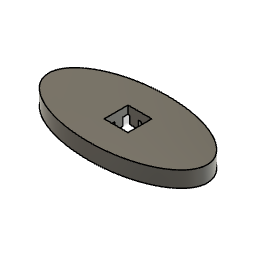
assy (Autodesk Fusion 360 archive; units mm, degrees)
design "cam gear"
Autodesk Fusion 360 part; units mm, degrees
sketch "Sketch1" plane through (0, 0, 0) normal (0, 1, 0) x (1, 0, 0)
  ellipse E0 centre (0, 0) end of major axis (10, 0) minor radius 5
  line L0 (-10, 0) -> (10, 0)
  line L1 (0, -5) -> (0, 5)
  line L2 (1.5, -1.5) -> (-1.5, -1.5)
  line L3 (-1.5, -1.5) -> (-1.5, 1.5)
  line L4 (-1.5, 1.5) -> (1.5, 1.5)
  line L5 (1.5, 1.5) -> (1.5, -1.5)
  line L6 (1.5, -1.5) -> (-1.5, 1.5) construction
  line L7 (-1.5, -1.5) -> (1.5, 1.5) construction
  dimension "d1" = 10
  dimension "d2" = 5
  dimension "d3" = 3
  dimension "d4" = 3
  constraint coincident E0.centre origin
  constraint horizontal L0
  constraint coincident E0 L0.start
  constraint coincident E0 L0.end
  constraint coincident E0 L1.start
  constraint coincident E0 L1.end
  constraint horizontal L2
  constraint perpendicular L2 L3
  constraint parallel L2 L4
  constraint parallel L3 L5
  constraint coincident L6 E0.centre
  constraint coincident L7 E0.centre
  measures "d1" distance of E0.centre L0.end
  measures "d2" distance of E0.centre L1.end
  measures "d3" distance of L3.end L4.end
  measures "d4" distance of L2.end L3.end
extrude "Extrude1" add sketch "Sketch1" along normal blind 2 contours E0 L0 L1 L4 L5 | E0 L0 L1 L2 L5 | E0 L0 L1 L3 L4 | E0 L0 L1 L2 L3 makes body 1
sketch "Sketch2" plane through (0, 0, 0) normal (0, -1, 0) x (1, 0, 0)
  line L0 (1.5, -1.5) -> (-1.5, -1.5)
  line L1 (-1.5, -1.5) -> (-1.5, 1.5)
  line L2 (-1.5, 1.5) -> (1.5, 1.5)
  line L3 (1.5, 1.5) -> (1.5, -1.5)
  ellipse E0 centre (0, 0) end of major axis (10, 0) minor radius 5 construction
  spline S0 degree 3 poles (-9, 0) (-9, -0.4805) (-8.7749, -1.0144) (-8.1755, -1.5893) (-7.3375, -2.3933) (-5.7684, -3.165) (-3.8472, -3.5923) (-1.5715, -4.0984) (1.1676, -4.1273) (3.4888, -3.6676) (5.2672, -3.3153) (6.7888, -2.6785) (7.7397, -1.9591) (8.5093, -1.3767) (8.8839, -0.7763) (8.9752, -0.2732) (9.0582, 0.1847) (8.958, 0.6291) (8.5638, 1.155) (8.019, 1.8817) (6.848, 2.6682) (5.2592, 3.2021) (3.1557, 3.9089) (0.3632, 4.1706) (-2.1616, 3.8753) (-4.2224, 3.6343) (-6.0882, 3.0261) (-7.3018, 2.261) (-8.2243, 1.6794) (-8.7451, 1.0304) (-8.9198, 0.492) (-8.9749, 0.3222) (-9, 0.1608) (-9, 0) knots -3.141593 -3.141593 -3.141593 -3.141593 -2.661128 -2.661128 -2.661128 -1.989339 -1.989339 -1.989339 -1.193608 -1.193608 -1.193608 -0.583919 -0.583919 -0.583919 -0.090453 -0.090453 -0.090453 0.358594 0.358594 0.358594 0.979103 0.979103 0.979103 1.800593 1.800593 1.800593 2.471093 2.471093 2.471093 2.980773 2.980773 2.980773 3.141593 3.141593 3.141593 3.141593
  line L4 (-0.5, 1.5) -> (-0.5, 3.9898)
  line L5 (0.5, 1.5) -> (0.5, 3.9898)
  line L6 (-1.079, 1.5) -> (-3.7306, 3.6146)
  line L7 (-1.4845, 0.5443) -> (-4.939, 3.2992)
  line L8 (-1.5, 0.1705) -> (-8.3644, -1.3963)
  line L9 (-1.5, -0.8552) -> (-7.3883, -2.1992)
  line L10 (-1.2773, -1.5) -> (-2.4053, -3.8422)
  line L11 (-0.1674, -1.5) -> (-1.3455, -3.9464)
  line L12 (0.1674, -1.5) -> (1.346, -3.9473)
  line L13 (1.2773, -1.5) -> (2.4058, -3.8432)
  line L14 (1.5, -0.8552) -> (7.3943, -2.2006)
  line L15 (1.5, 0.1705) -> (8.3629, -1.3959)
  line L16 (1.4845, 0.5443) -> (4.9439, 3.3031)
  line L17 (1.079, 1.5) -> (3.7295, 3.6137)
  dimension "d7" = -1
  constraint coincident L2 L4.start
  constraint coincident S0 L4.end
  constraint perpendicular L2 L4
  constraint coincident S0 L6.end
  constraint coincident S0 L7.end
  constraint coincident S0 L8.end
  constraint coincident S0 L10.end
  constraint coincident S0 L11.end
  constraint coincident S0 L9.end
  constraint coincident S0 L12.end
  constraint coincident S0 L13.end
  constraint coincident S0 L14.end
  constraint coincident S0 L15.end
  constraint coincident S0 L16.end
  constraint coincident S0 L17.end
  constraint coincident L1 L9.start
  constraint coincident L2 L6.start
  constraint coincident L2 L17.start
  constraint coincident L3 L14.start
  constraint coincident L0 L13.start
  constraint coincident L0 L10.start
  constraint coincident L1 L8.start
  constraint coincident L0 L11.start
  constraint coincident L0 L12.start
  constraint coincident L3 L15.start
extrude "Extrude2" cut sketch "Sketch2" against normal blind 1 contours L0 L3 S0 L13 L14 | L0 S0 L11 L12 | L3 S0 L15 L16 | L0 L1 S0 L9 L10 | L2 S0 L5 L17 | L1 S0 L7 L8 | L2 S0 L4 L6 bodies 1
copy_body "Body->Comp1" bodies 1 removing the originals makes body 2 in component "Component"
component "Component" placed x (1, 0, 0) y (0, 1, 0) z (0, 0, 1) at (0, 0, 0)

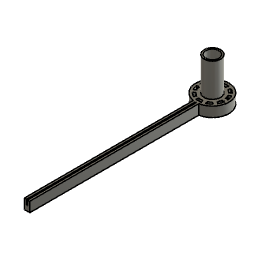
design "reciprocator"
Autodesk Fusion 360 part; units mm, degrees
sketch "Sketch1" plane through (0, 0, 0) normal (0, 1, 0) x (1, 0, 0)
  circle A0 centre (0, 0) radius 5
  circle A1 centre (0, 0) radius 2.5
  line L0 (-4.9749, -0.5) -> (-4.9749, 0.5)
  line L1 (4.9749, 0.5) -> (4.9749, -0.5)
  line L2 (-4.9749, 0.5) -> (-3.4641, 0.5)
  line L3 (3.4641, 0.5) -> (4.9749, 0.5)
  line L4 (4.9749, -0.5) -> (3.4641, -0.5)
  line L5 (-3.4641, -0.5) -> (-4.9749, -0.5)
  circle A2 centre (0, 0) radius 3.5
  line L6 (-0.5949, -3.4491) -> (-1.0618, -4.886)
  line L7 (-2.0129, -4.5769) -> (-1.546, -3.14)
  line L8 (2.0129, 4.5769) -> (1.546, 3.14)
  line L9 (0.5949, 3.4491) -> (1.0618, 4.886)
  line L10 (3.0964, -1.6316) -> (4.3187, -2.5197)
  line L11 (3.7309, -3.3287) -> (2.5086, -2.4407)
  line L12 (-3.7309, 3.3287) -> (-2.5086, 2.4407)
  line L13 (-3.0964, 1.6316) -> (-4.3187, 2.5197)
  line L14 (2.5086, 2.4407) -> (3.7309, 3.3287)
  line L15 (4.3187, 2.5197) -> (3.0964, 1.6316)
  line L16 (-4.3187, -2.5197) -> (-3.0964, -1.6316)
  line L17 (-2.5086, -2.4407) -> (-3.7309, -3.3287)
  line L18 (-1.546, 3.14) -> (-2.0129, 4.5769)
  line L19 (-1.0618, 4.886) -> (-0.5949, 3.4491)
  line L20 (1.0618, -4.886) -> (0.5949, -3.4491)
  line L21 (1.546, -3.14) -> (2.0129, -4.5769)
  arc A3 (-1.7794, 3.8585) -> (-3.1198, 2.8847) centre (0, 0) ccw
  arc A4 (-3.7076, 2.0757) -> (-4.2195, 0.5) centre (0, 0) ccw
  arc A5 (-4.2195, -0.5) -> (-3.7076, -2.0757) centre (0, 0) ccw
  arc A6 (-3.1198, -2.8847) -> (-1.7794, -3.8585) centre (0, 0) ccw
  arc A7 (-0.8284, -4.1675) -> (0.8284, -4.1675) centre (0, 0) ccw
  arc A8 (1.7794, -3.8585) -> (3.1198, -2.8847) centre (0, 0) ccw
  arc A9 (3.7076, -2.0757) -> (4.2195, -0.5) centre (0, 0) ccw
  arc A10 (4.2195, 0.5) -> (3.7076, 2.0757) centre (0, 0) ccw
  arc A11 (3.1198, 2.8847) -> (1.7794, 3.8585) centre (0, 0) ccw
  arc A12 (0.8284, 4.1675) -> (-0.8284, 4.1675) centre (0, 0) ccw
  line L22 (-0.8284, -5.9767) -> (-0.8284, -4.9309)
  line L23 (0.8284, -4.9309) -> (0.8284, -5.9767)
  line L24 (0.8284, -5.9767) -> (0.8284, -55.9767)
  line L25 (-0.8284, -5.9767) -> (-0.8284, -55.9767)
  line L26 (0.8284, -55.9767) -> (-0.8284, -55.9767)
  line L27 (0.1716, -5.9767) -> (0.1716, -55.9767)
  line L28 (0.1716, -5.9767) -> (0.1716, -4.9309)
  line L29 (-0.1716, -4.9309) -> (-0.1716, -5.9767)
  line L30 (-0.1716, -5.9767) -> (-0.1716, -55.9767)
  dimension "d1" = 10
  dimension "d2" = 5
  dimension "d10" = 1
  dimension "d11" = 1
  dimension "d13" = 360
  dimension "d16" = 1.0458
  dimension "d17" = 50
  dimension "d18" = 50
  constraint concentric A0 A1
  constraint horizontal L4
  constraint perpendicular L0 L4
  constraint parallel L2 L4
  constraint parallel L0 L1
  constraint coincident A0 L1.end
  constraint coincident A0.centre A1.centre
  constraint collinear L2 L3
  constraint collinear L4 L5
  constraint concentric A1 A2
  constraint coincident A2 L2.end
  constraint coincident A2 L5.start
  constraint coincident A2 L4.end
  constraint coincident A2 L3.start
  constraint concentric A1 A3
  constraint coincident L19 A12.end
  constraint coincident L18 A3.start
  constraint coincident L12 A3.end
  constraint coincident L13 A4.start
  constraint concentric A3 A4
  constraint coincident L2 A4.end
  constraint coincident L5 A5.start
  constraint concentric A4 A5
  constraint coincident L16 A5.end
  constraint coincident L17 A6.start
  constraint concentric A5 A6
  constraint coincident L7 A6.end
  constraint coincident L6 A7.start
  constraint concentric A6 A7
  constraint coincident L20 A7.end
  constraint coincident L21 A8.start
  constraint concentric A7 A8
  constraint coincident L11 A8.end
  constraint coincident L10 A9.start
  constraint concentric A8 A9
  constraint coincident L4 A9.end
  constraint coincident L3 A10.start
  constraint concentric A9 A10
  constraint coincident L15 A10.end
  constraint coincident L14 A11.start
  constraint concentric A10 A11
  constraint coincident L8 A11.end
  constraint coincident L9 A12.start
  constraint concentric A11 A12
  constraint parallel L22 L23
  constraint coincident A0 L23.start
  constraint coincident A0 L22.end
  constraint parallel L23 L24
  constraint parallel L22 L25
  constraint perpendicular L25 L26
  constraint parallel L25 L27
  constraint parallel L22 L28
  constraint parallel L23 L29
  constraint parallel L24 L30
  constraint coincident L26 L27.end
  constraint coincident L26 L30.end
  measures "d1" diameter of A0
  measures "d2" diameter of A1
  measures "d10" distance of L2 L4
  measures "d11" distance of A1 A2
  measures "d16" distance of L23.end L23.start
  measures "d17" distance of L23.end L24.end
  measures "d18" distance of L22.start L25.end
extrude "Extrude1" add sketch "Sketch1" along normal blind 10 contours A1 makes body 1
extrude "Extrude2" add sketch "Sketch1" against normal blind 3 separate body contours A0 L1 | A0 L3 L15 A10 | L1 L3 L4 A2 | A0 L4 L10 A9 | A0 A2 L14 L15 | L3 A2 L15 A10 | A0 A2 L10 L11 | L4 A2 L10 A9 | A0 L8 L14 A11 | A2 | A0 L11 L21 A8 | A0 A2 L8 L9 | A2 L8 L14 A11 | A0 A2 L20 L21 | A2 L11 L21 A8 | A0 L9 L19 A12 | A0 L6 L20 A7 | A0 A2 L18 L19 | A2 L9 L19 A12 | A2 L6 L20 A7 | A0 L12 L18 A3 | A0 A2 L6 L7 | A0 A2 L12 L13 | A2 L12 L18 A3 | A0 L2 L13 A4 | A2 L7 L17 A6 | A0 L7 L17 A6 | A0 L0 | L0 L2 L5 A2 | L2 A2 L13 A4 | A0 A2 L16 L17 | A0 L5 L16 A5 | L5 A2 L16 A5 makes body 2
sketch "Sketch2" plane through (0, 10, 0) normal (0, 1, 0) x (-1, 0, 0)
  circle A0 centre (0, 0) radius 2.5
  circle A1 centre (0, 0) radius 2
  dimension "d7" = 4
  constraint coincident A0.centre A1.centre
  measures "d7" diameter of A1
extrude "Extrude3" cut sketch "Sketch2" against normal blind 9 contours A1 bodies 1
extrude "Extrude4" cut sketch "Sketch1" against normal blind 3 contours L3 A2 L15 A10 | L4 A2 L10 A9 | A2 L8 L14 A11 | A2 L11 L21 A8 | A2 L9 L19 A12 | A2 L6 L20 A7 | A2 L12 L18 A3 | A2 L7 L17 A6 | L2 A2 L13 A4 | L5 A2 L16 A5 bodies 2
extrude "Extrude5" add sketch "Sketch1" against normal blind 3 contours A0 L23 L24 L26 L27 L28 | A0 L26 L27 L28 L29 L30 | A0 L22 L25 L26 L29 L30 bodies 2
extrude "Extrude6" cut sketch "Sketch1" against normal blind 1.5 contours A0 L26 L27 L28 L29 L30 bodies 2
combine "Combine1" operation add target body 2 tool bodies 1
copy_body "Body->Comp3" bodies 2 removing the originals makes body 3 in component "Component"
component "Component" placed x (1, 0, 0) y (0, 1, 0) z (0, 0, 1) at (0, 0, 0)

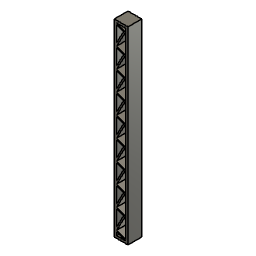
design "spindle"
Autodesk Fusion 360 part; units mm, degrees
sketch "Sketch1" plane through (0, 0, 0) normal (0, 1, 0) x (1, 0, 0)
  line L0 (1.45, -1.45) -> (-1.45, -1.45)
  line L1 (-1.45, -1.45) -> (-1.45, 1.45)
  line L2 (-1.45, 1.45) -> (1.45, 1.45)
  line L3 (1.45, 1.45) -> (1.45, -1.45)
  line L4 (1.45, -1.45) -> (-1.45, 1.45) construction
  line L5 (-1.45, -1.45) -> (1.45, 1.45) construction
  dimension "d1" = 2.9
  dimension "d2" = 2.9
  constraint horizontal L0
  constraint perpendicular L0 L1
  constraint parallel L0 L2
  constraint parallel L1 L3
  constraint coincident L4 origin
  constraint coincident L5 origin
  measures "d1" distance of L0.start L2.end
  measures "d2" distance of L1.end L2.end
extrude "Extrude1" add sketch "Sketch1" along normal blind 40 makes body 1
sketch "Sketch2" plane through (0, 0, 1.45) normal (0, 0, 1) x (1, 0, 0)
  line L0 (-1.45, 0) -> (1.45, 0)
  line L1 (1.45, 0) -> (1.45, 40)
  line L2 (1.45, 40) -> (-1.45, 40)
  line L3 (-1.45, 40) -> (-1.45, 0)
  line L4 (-0.95, 39.5) -> (-0.95, 0.5)
  line L5 (-0.95, 0.5) -> (0.95, 0.5)
  line L6 (0.95, 0.5) -> (0.95, 39.5)
  line L7 (0.95, 39.5) -> (-0.95, 39.5)
  line L8 (-0.95, 39.5) -> (0.95, 38.8085)
  line L9 (-0.95, 35.2778) -> (0.95, 34.5862)
  line L10 (-0.95, 31.0556) -> (0.95, 30.364)
  line L11 (-0.95, 26.8333) -> (0.95, 26.1418)
  line L12 (-0.95, 22.6111) -> (0.95, 21.9196)
  line L13 (-0.95, 18.3889) -> (0.95, 17.6973)
  line L14 (-0.95, 14.1667) -> (0.95, 13.4751)
  line L15 (-0.95, 9.9444) -> (0.95, 9.2529)
  line L16 (-0.95, 5.7222) -> (0.95, 5.0307)
  line L17 (-0.95, 1.5) -> (0.95, 0.8085)
  line L18 (0.95, 38.8085) -> (-0.95, 35.2778)
  line L19 (0.95, 34.5862) -> (-0.95, 31.0556)
  line L20 (0.95, 30.364) -> (-0.95, 26.8333)
  line L21 (0.95, 26.1418) -> (-0.95, 22.6111)
  line L22 (0.95, 21.9196) -> (-0.95, 18.3889)
  line L23 (0.95, 17.6973) -> (-0.95, 14.1667)
  line L24 (0.95, 13.4751) -> (-0.95, 9.9444)
  line L25 (0.95, 9.2529) -> (-0.95, 5.7222)
  line L26 (0.95, 5.0307) -> (-0.95, 1.5)
  line L27 (-1.0526, 39.2181) -> (0.5215, 38.6452)
  line L28 (0.5215, 38.6452) -> (-1.3785, 35.1145)
  line L29 (-1.3785, 35.1145) -> (0.5215, 34.423)
  line L30 (0.5215, 34.423) -> (-1.3785, 30.8923)
  line L31 (-1.3785, 30.8923) -> (0.5215, 30.2007)
  line L32 (0.5215, 30.2007) -> (-1.3785, 26.6701)
  line L33 (-1.3785, 26.6701) -> (0.5215, 25.9785)
  line L34 (0.5215, 25.9785) -> (-1.3785, 22.4478)
  line L35 (-1.3785, 22.4478) -> (0.5215, 21.7563)
  line L36 (0.5215, 21.7563) -> (-1.3785, 18.2256)
  line L37 (-1.3785, 18.2256) -> (0.5215, 17.5341)
  line L38 (0.5215, 17.5341) -> (-1.3785, 14.0034)
  line L39 (-1.3785, 14.0034) -> (0.5215, 13.3118)
  line L40 (0.5215, 13.3118) -> (-1.3785, 9.7812)
  line L41 (-1.3785, 9.7812) -> (0.5215, 9.0896)
  line L42 (0.5215, 9.0896) -> (-1.3785, 5.5589)
  line L43 (-1.3785, 5.5589) -> (0.5215, 4.8674)
  line L44 (0.5215, 4.8674) -> (-1.3785, 1.3367)
  line L45 (-1.3785, 1.3367) -> (0.9203, 0.5)
  dimension "d5" = -0.5
  dimension "d6" = 70
  dimension "d9" = -38
  dimension "d10" = 0
  constraint coincident L6 L8.end
  constraint parallel L8 L27
  constraint parallel L18 L28
  constraint parallel L9 L29
  constraint parallel L19 L30
  constraint parallel L10 L31
  constraint parallel L20 L32
  constraint parallel L11 L33
  constraint parallel L21 L34
  constraint parallel L12 L35
  constraint parallel L22 L36
  constraint parallel L13 L37
  constraint parallel L23 L38
  constraint parallel L14 L39
  constraint parallel L24 L40
  constraint parallel L15 L41
  constraint parallel L25 L42
  constraint parallel L16 L43
  constraint parallel L26 L44
  constraint parallel L17 L45
  constraint coincident L5 L45.end
  measures "d6" angle of L4 L8
extrude "Extrude2" cut sketch "Sketch2" against normal blind 2 contours L6 L7 L8 | L4 L27 L28 | L6 L9 L18 | L6 L10 L19 | L6 L11 L20 | L4 L29 L30 | L6 L12 L21 | L4 L31 L32 | L6 L13 L22 | L4 L33 L34 | L6 L14 L23 | L4 L35 L36 | L6 L15 L24 | L4 L37 L38 | L6 L16 L25 | L4 L39 L40 | L6 L17 L26 | L4 L41 L42 | L4 L43 L44 | L4 L5 L45 bodies 1
copy_body "Body->Comp1" bodies 1 removing the originals makes body 2 in component "Component"
component "Component" placed x (1, 0, 0) y (0, 1, 0) z (0, 0, 1) at (0, 0, 0)

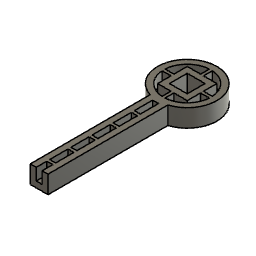
design "lever"
Autodesk Fusion 360 part; units mm, degrees
sketch "Sketch1" plane through (0, 0, 0) normal (0, 1, 0) x (1, 0, 0)
  circle A0 centre (0, 0) radius 5
  line L0 (1.5, -1.5) -> (-1.5, -1.5)
  line L1 (-1.5, -1.5) -> (-1.5, 1.5)
  line L2 (-1.5, 1.5) -> (1.5, 1.5)
  line L3 (1.5, 1.5) -> (1.5, -1.5)
  line L4 (1.5, -1.5) -> (-1.5, 1.5) construction
  line L5 (-1.5, -1.5) -> (1.5, 1.5) construction
  line L6 (0, 0) -> (0, -5) construction
  line L7 (1.5, -35) -> (-1.5, -35)
  line L8 (-1.5, 25) -> (1.5, 25)
  line L9 (0, -5) -> (-0.4988, 4.9751) construction
  line L10 (0, -5) -> (0.4988, 4.9751) construction
  line L11 (1.5, 1.5) -> (1.5, -1.5)
  line L12 (1.5, -4.7697) -> (1.5, -35)
  line L13 (-1.5, -35) -> (-1.5, -4.7697)
  line L14 (-1.5, -1.5) -> (-1.5, 1.5)
  dimension "d1" = 10
  dimension "d2" = 3
  dimension "d3" = 3
  dimension "d4" = 3
  dimension "d5" = 30
  constraint coincident A0.centre L6.start
  constraint horizontal L0
  constraint perpendicular L0 L1
  constraint parallel L0 L2
  constraint parallel L1 L3
  constraint coincident L4 A0.centre
  constraint coincident L5 A0.centre
  constraint perpendicular L0 L6
  constraint horizontal L7
  constraint perpendicular L7 L13
  constraint parallel L7 L8
  constraint parallel L11 L13
  constraint coincident A0 L6.end
  constraint coincident A0 L10.end
  constraint coincident A0 L9.end
  constraint coincident A0 L12.start
  constraint collinear L11 L12
  constraint coincident A0 L13.end
  constraint collinear L13 L14
  measures "d1" diameter of A0
  measures "d2" distance of L1.end L2.end
  measures "d3" distance of L0.start L2.end
  measures "d4" distance of L7.start L7.end
  measures "d5" distance of L7 L6.end
extrude "Extrude1" add sketch "Sketch1" along normal blind 3
sketch "Sketch2" plane through (0, 3, 0) normal (0, 1, 0) x (-1, 0, 0)
  line L0 (-1.5, 1.5) -> (1.5, 1.5)
  line L1 (1.5, 1.5) -> (1.5, -1.5)
  line L2 (1.5, -1.5) -> (-1.5, -1.5)
  line L3 (-1.5, -1.5) -> (-1.5, 1.5)
  arc A0 (-1.5, 4.7697) -> (1.5, 4.7697) centre (0, 0) ccw
  line L4 (1.5, 4.7697) -> (1.5, 35)
  line L5 (1.5, 35) -> (-1.5, 35)
  line L6 (-1.5, 35) -> (-1.5, 4.7697)
  line L7 (0.5, 34) -> (-0.5, 34)
  line L8 (-0.5, 34) -> (-0.5, 3.9686)
  arc A1 (0, 4) -> (0.2464, 3.9924) centre (0, 0) ccw
  line L9 (0.5, 3.9686) -> (0.5, 34)
  line L10 (-2.5, -2.5) -> (-2.5, 2.5)
  line L11 (-2.5, 2.5) -> (2.5, 2.5)
  line L12 (2.5, 2.5) -> (2.5, -2.5)
  line L13 (2.5, -2.5) -> (-2.5, -2.5)
  line L14 (-0.2536, -2.5) -> (-0.2536, -4)
  line L15 (0, -4) -> (0, -2.5) construction
  line L16 (0, -1.5) -> (0, 4.8511) construction
  line L17 (-0.2536, -4) -> (0, -2.5) construction
  line L18 (0.2464, -4) -> (0, -2.5) construction
  line L19 (0.2464, -4) -> (0.2464, -2.5)
  line L20 (2.5, -0.2536) -> (4, -0.2536)
  line L21 (4, 0.2464) -> (2.5, 0.2464)
  line L22 (0.2536, 2.5) -> (0.2536, 4)
  line L23 (-0.2464, 4) -> (-0.2464, 2.5)
  line L24 (-2.5, 0.2536) -> (-4, 0.2536)
  line L25 (-4, -0.2464) -> (-2.5, -0.2464)
  line L26 (0.5, 4.8511) -> (-0.5, 4.8511)
  line L27 (0.5, 5.3511) -> (-0.5, 5.3511)
  line L28 (0.5, 8.9225) -> (-0.5, 8.9225)
  line L29 (0.5, 8.4225) -> (-0.5, 8.4225)
  line L30 (0.5, 12.4939) -> (-0.5, 12.4939)
  line L31 (0.5, 11.9939) -> (-0.5, 11.9939)
  line L32 (0.5, 16.0654) -> (-0.5, 16.0654)
  line L33 (0.5, 15.5654) -> (-0.5, 15.5654)
  line L34 (0.5, 19.6368) -> (-0.5, 19.6368)
  line L35 (0.5, 19.1368) -> (-0.5, 19.1368)
  line L36 (0.5, 23.2082) -> (-0.5, 23.2082)
  line L37 (0.5, 22.7082) -> (-0.5, 22.7082)
  line L38 (0.5, 26.7796) -> (-0.5, 26.7796)
  line L39 (0.5, 26.2796) -> (-0.5, 26.2796)
  line L40 (0.5, 30.3511) -> (-0.5, 30.3511)
  line L41 (0.5, 29.8511) -> (-0.5, 29.8511)
  dimension "d9" = -1
  dimension "d12" = 0.5
  dimension "d14" = 360
  dimension "d15" = 0.5
  dimension "d18" = 0
  dimension "d19" = 0
  dimension "d22" = 25
  dimension "d23" = 0
  constraint perpendicular L11 L15
  constraint midpoint L13 L15.end
  constraint coincident L13 L14.start
  constraint coincident L2 L16.start
  constraint collinear L15 L16
  constraint coincident L13 L19.end
  constraint parallel L5 L7
  constraint parallel L6 L8
  constraint concentric A0 A1
  constraint parallel L4 L9
  constraint coincident A1 L15.start
  constraint coincident L9.start A1
  constraint coincident L8.end A1
  constraint coincident L9 L26.start
  constraint coincident L8 L26.end
  constraint perpendicular L8 L26
  constraint coincident L9 L27.start
  constraint coincident L8 L27.end
  constraint perpendicular L8 L27
  measures "d12" distance of L14 L19
  measures "d15" distance of L26 L27
extrude "Extrude3" cut sketch "Sketch2" against normal blind 2 contours L7 L8 L9 L40 | L8 L9 L38 L41 | L8 L9 L36 L39 | L8 L9 L34 L37 | L8 L9 L32 L35 | L8 L9 L30 L33 | L8 L9 L28 L31 | L8 L9 L27 L29 | A1 L11 L12 L21 L22 | A1 L10 L11 L23 L24 | A1 L12 L13 L19 L20 | A1 L10 L13 L14 L25
extrude "Extrude2" cut sketch "Sketch2" against normal blind 2 contours L7 L8 L9 L40 | L8 L9 L40 L41 | L8 L9 L38 L41 | L8 L9 L38 L39 | L8 L9 L36 L39 | L8 L9 L36 L37 | L8 L9 L34 L37 | L8 L9 L34 L35 | L8 L9 L32 L35 | L8 L9 L32 L33 | L8 L9 L30 L33 | L8 L9 L30 L31 | L8 L9 L28 L31 | L8 L9 L28 L29 | L8 L9 L27 L29 | L8 L9 L26 L27 | L8 A1 L9 L11 L22 L23 L26 | A1 L11 L12 L21 L22 | A1 L10 L11 L23 L24 | A1 L12 L20 L21 | A1 L10 L24 L25 | A1 L12 L13 L19 L20 | A1 L10 L13 L14 L25 | A1 L13 L14 L19
extrude "Extrude4" add sketch "Sketch2" against normal blind 2 contours L8 L9 L40 L41 | L8 L9 L38 L39 | L8 L9 L36 L37 | L8 L9 L34 L35 | L8 L9 L32 L33 | L8 L9 L30 L31 | L8 L9 L28 L29 | L8 L9 L26 L27 | A1 L12 L20 L21 | A1 L10 L24 L25 | A1 L13 L14 L19
extrude "Extrude5" cut 1 faces at (-0.5, 2, 35) along direction (0, 0, -1) blind 10
extrude "Extrude6" add sketch "Sketch2" against normal blind 2 contours L8 A1 L9 L11 L22 L23 L26

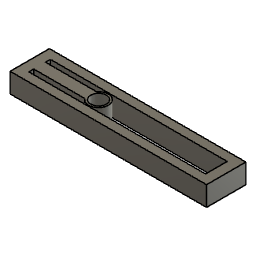
design "guide"
Autodesk Fusion 360 part; units mm, degrees
sketch "Sketch1" plane through (0, 0, 0) normal (0, 1, 0) x (1, 0, 0)
  line L0 (25, -5) -> (-25, -5)
  line L1 (-25, -5) -> (-25, 5)
  line L2 (-25, 5) -> (25, 5)
  line L3 (25, 5) -> (25, -5)
  line L4 (22.5, 2.75) -> (-22.5, 2.75)
  line L5 (-22.5, -2.75) -> (22.5, -2.75)
  line L6 (22.5, -2.75) -> (22.5, 2.75)
  line L7 (-25, 0) -> (-15.3523, 0) construction
  line L8 (-22.5, 2.75) -> (-22.5, 1.5)
  line L9 (-22.5, -1.5) -> (-22.5, -2.75)
  arc A0 (-9.5, -1.5) -> (-9.5, 1.5) centre (-7.5, 0) ccw
  line L10 (-22.5, 1.5) -> (-9.5, 1.5)
  line L11 (-22.5, -1.5) -> (-9.5, -1.5)
  circle A1 centre (-7.5, 0) radius 2
  dimension "d1" = 10
  dimension "d2" = 5.5
  dimension "d3" = 50
  dimension "d4" = 45
  dimension "d5" = 1.5
  dimension "d7" = 5
  dimension "d8" = 4
  constraint horizontal L0
  constraint perpendicular L0 L1
  constraint parallel L0 L2
  constraint parallel L1 L3
  constraint horizontal L4
  constraint perpendicular L4 L8
  constraint parallel L4 L5
  constraint parallel L6 L8
  constraint midpoint L1 L7.start
  constraint perpendicular L7 L8
  constraint perpendicular L8 L10
  constraint symmetric L7 L8.end L9.start
  constraint collinear L8 L9
  constraint concentric A0 A1
  measures "d1" distance of L0.end L1.end
  measures "d2" distance of L4.end L5.start
  measures "d3" distance of L1.end L2.end
  measures "d4" distance of L4.start L4.end
  measures "d5" distance of L7.end L10
  measures "d7" diameter of A0
  measures "d8" diameter of A1
extrude "Extrude1" add sketch "Sketch1" along normal blind 5 makes body 1
copy_body "Body->Comp1" bodies 1 removing the originals makes body 2 in component "Component"
component "Component" placed x (1, 0, 0) y (0, 1, 0) z (0, 0, 1) at (0, 0, 0)

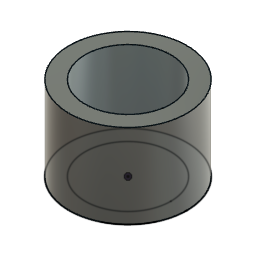
design "recipro cap"
Autodesk Fusion 360 part; units mm, degrees
sketch "Sketch1" plane through (0, 0, 0) normal (0, 1, 0) x (1, 0, 0)
  circle A0 centre (0, 0) radius 3.5
  circle A1 centre (0, 0) radius 2.55
  dimension "d1" = 7
  dimension "d2" = 5.1
  constraint coincident A0.centre A1.centre
  measures "d1" diameter of A0
  measures "d2" diameter of A1
extrude "Extrude1" add sketch "Sketch1" along normal blind 5 makes body 1
extrude "Extrude2" add sketch "Sketch1" along normal blind 1 contours A1 bodies 1
sketch "Sketch2" plane through (0, 5, 0) normal (0, 1, 0) x (-1, 0, 0)
  circle A0 centre (0, 0) radius 2.55
  circle A1 centre (0, 0) radius 3.5
copy_body "Body->Comp1" bodies 1 removing the originals makes body 2 in component "Component"
component "Component" placed x (1, 0, 0) y (0, 1, 0) z (0, 0, 1) at (0, 0, 0)
